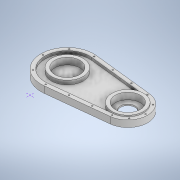
# Autodesk Inventor part: Abdeckung
Saved by Autodesk Inventor 2021 (Build 250183000, 183)
## iProperties
Created: 2021-01-19
Part Number: Abdeckung
Material: Generisch
Document SubType Name: Modeling
Designer: Jaro Machnow
Density: 1 g/cm^3
Appearance: Vorgabe
Author: Jaro Machnow
Autodesk Inventor part; units mm, degrees
ref_plane "YZ Plane" through (0, 0, 0) normal (1, 0, 0) x (0, 1, 0)
ref_plane "XZ Plane" through (0, 0, 0) normal (0, 1, 0) x (-1, 0, 0)
ref_plane "XY Plane" through (0, 0, 0) normal (0, 0, 1) x (1, 0, 0)
sketch "Skizze7" plane through (0, 0, 0) normal (0, -1, 0) x (1, 0, 0)
  point P0 (-1.84433, 26.478034)
sketch "Skizze1" plane through (0, 0, 0) normal (0, 1, 0) x (-1, 0, 0)
  arc A0 (-2.173913, -19.881502) -> (-2.173913, 19.881502) centre (0, 0) ccw
  arc A1 (-47.630435, 14.911126) -> (-47.630435, -14.911126) centre (-46, 0) ccw
  line L0 (-2.173913, 19.881502) -> (-47.630435, 14.911126)
  line L1 (-2.173913, -19.881502) -> (-47.630435, -14.911126)
  line L2 (45.02348, 0) -> (-115.148005, 0) construction
  dimension "d0" = 40
  dimension "d1" = 30
  dimension "d2" = 46
  constraints: 6 end point, 4 point on circle, 4 tangent, 2 centre point, 2 horizontal, 1 coincident, 1 point on line
  measures "d0" diameter of A0
  measures "d1" diameter of A1
  measures "d2" distance of A1.centre point (0, 0)
extrude "Extrusion1" add sketch "Skizze1" along normal blind 5
shell "Wandung1" thickness 3 removed faces 1 at (17.326087, 5, -4.970375)
sketch "Skizze2" plane through (0, 3, 0) normal (0, 1, 0) x (1, 0, 0)
  circle A0 centre (0, 0) radius 9.5
  circle A1 centre (0, 0) radius 12
  dimension "d6" = 19
  dimension "d7" = 24
  constraints: 2 centre point, 2 coincident
  measures "d6" diameter of A0
  measures "d7" diameter of A1
extrude "Extrusion2" add sketch "Skizze2" along normal blind 3
sketch "Skizze3" plane through (0, 3, 0) normal (0, 1, 0) x (1, 0, 0)
  arc A0 (47.304348, -11.928901) -> (47.304348, 11.928901) centre (46, 0) ccw
  circle A1 centre (46, 0) radius 9.5
  circle A2 centre (46, 0) radius 12
  point P0 (0, 0)
  point P1 (47.304348, -11.928901)
  dimension "d10" = 19
  constraints: 2 centre point, 2 coincident
  measures "d10" diameter of A1
extrude "Extrusion3" add sketch "Skizze3" along normal blind 3
sketch "Skizze4" plane through (0, 3, 0) normal (0, 1, 0) x (1, 0, 0)
  circle A0 centre (0, 0) radius 9.5
  constraints: 1 centre point, 1 coincident
extrude "Extrusion4" cut sketch "Skizze4" against normal blind 2
sketch "Skizze5" plane through (46, 3, 0) normal (0, 1, 0) x (1, 0, 0)
  circle A0 centre (0, 0) radius 9.5
  point P0 (-46, 0)
  constraints: 1 centre point
extrude "Extrusion5" cut sketch "Skizze5" against normal blind 2
sketch "Skizze6" plane through (46, 1, 0) normal (0, 1, 0) x (1, 0, 0)
  point P0 (-46, 0)
  point P1 (0, 0)
  point P2 (0, 0)
  constraints: 1 coincident
hole "Bohrung1" at (46, 1, 0) direction (0, -1, 0) diameter 11 end through all
sketch "Skizze8" plane through (0, 5, 0) normal (0, 1, 0) x (1, 0, 0)
  arc A0 (1.847826, 16.899276) -> (1.847826, -16.899276) centre (0, 0) ccw
  arc A1 (2.173913, 19.881502) -> (2.173913, -19.881502) centre (0, 0) ccw
  line L0 (47.304348, -11.928901) -> (1.847826, -16.899276)
  line L1 (2.173913, -19.881502) -> (47.630435, -14.911126)
  arc A2 (47.630435, -14.911126) -> (47.630435, 14.911126) centre (46, 0) ccw
  circle A3 centre (46, 0) radius 12
  line L2 (1.847826, 16.899276) -> (47.304348, 11.928901)
  line L3 (47.630435, 14.911126) -> (2.173913, 19.881502)
  arc A4 (2.01087, 18.390389) -> (2.01087, -18.390389) centre (0, 0) ccw
  line L4 (2.01087, 18.390389) -> (47.467391, 13.420014)
  arc A5 (47.467391, -13.420014) -> (47.467391, 13.420014) centre (46, 0) ccw
  line L5 (47.467391, -13.420014) -> (2.01087, -18.390389)
  line L6 (47.467391, 13.420014) -> (46, 0) construction
  line L7 (46, 0) -> (47.467391, -13.420014) construction
  line L8 (0, 0) -> (2.01087, -18.390389) construction
  line L9 (0, 0) -> (2.01087, 18.390389) construction
  point P0 (0, -18.5)
  point P1 (56.051373, -9.012208)
  point P2 (59.5, 0.000031)
  point P3 (56.051332, 9.012254)
  point P4 (47.46733, 13.42002)
  point P5 (-12.350063, -13.774104)
  point P6 (-18.5, -0.000042)
  point P7 (-12.350126, 13.774047)
  point P8 (2.010785, 18.390398)
  point P9 (17.916071, -16.651258)
  point P10 (33.821272, -14.912128)
  point P11 (17.916071, 16.651258)
  point P12 (17.915987, 16.651268)
  point P13 (33.821272, 14.912128)
  point P14 (33.821188, 14.912137)
  dimension "d24" = 1.5
  dimension "d26" = 167.52
  dimension "d29" = 167.52
  dimension "d31" = 167.52
  dimension "d34" = 192.48
  dimension "d38" = 16
  dimension "d45" = 16
  constraints: 12 end point, 6 point on circle, 2 centre point, 1 coincident, 21 other
  measures "d24" radial gap between concentric circles of A1 A4
  measures "d26" angle of L7 L6
  measures "d31" angle of L9 L8
  measures "d38" distance of point (2.011, -18.39) point (17.916, -16.651)
  measures "d45" distance of L4.start point (17.916, 16.651)
hole "Bohrung2" at (2.01087, 5, 18.390389) at (-12.350063, 5, 13.774104) at (-18.5, 5, 0.000042) at (-12.350126, 5, -13.774047) at (2.010785, 5, -18.390398) at (17.915987, 5, -16.651268) at (33.821272, 5, -14.912128) at (47.46733, 5, -13.42002) at (56.051332, 5, -9.012254) at (59.5, 5, -0.000031) at (56.051373, 5, 9.012208) at (47.467391, 5, 13.420014) at (33.821272, 5, 14.912128) at (17.916071, 5, 16.651258) direction (0, -1, 0) diameter 1 end through all
